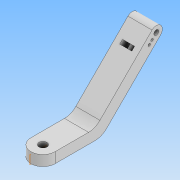
# Autodesk Inventor part: 主吊臂
Saved by Autodesk Inventor 2021 (Build 250183000, 183)
## iProperties
Created: 2025-12-12
Part Number: 主吊臂
Material: 一般
Document SubType Name: Modeling
Designer: User
Density: 1 g/cm^3
Appearance: 預設
Author: User
Autodesk Inventor part; units mm, degrees
ref_plane "YZ Plane" through (0, 0, 0) normal (1, 0, 0) x (0, 1, 0)
ref_plane "XZ Plane" through (0, 0, 0) normal (0, 1, 0) x (-1, 0, 0)
ref_plane "XY Plane" through (0, 0, 0) normal (0, 0, 1) x (1, 0, 0)
sketch "草圖1" plane through (0, 0, 0) normal (0, 1, 0) x (-1, 0, 0)
  line L0 (0, 150) -> (-300, 150)
  line L1 (-300, 0) -> (-300, 150)
  arc A0 (-300, 0) -> (0, 0) centre (-150, 0) ccw
  line L2 (0, 150) -> (0, 0)
  line L3 (0, 271.7864) -> (0, 150)
  line L4 (-300, 271.7864) -> (0, 271.7864)
  line L5 (-300, 150) -> (-300, 271.7864)
  circle A1 centre (-150, 0) radius 50
  line L6 (-30.3819, -276.523) -> (-200, -276.523)
  line L7 (0, -703.0461) -> (-300, -703.0461)
  line L8 (-300, -553.0461) -> (-300, -703.0461)
  arc A2 (0, -553.0461) -> (-300, -553.0461) centre (-150, -553.0461) ccw
  line L9 (0, -703.0461) -> (0, -553.0461)
  circle A3 centre (-150, -553.0461) radius 50
  constraints: 20 end point, 7 symmetric about line, 4 centre point, 4 point on circle, 1 horizontal, 2 other
extrude "擠出1" add sketch "草圖1" along normal blind 130 contours L7 L8 A2 L9
ref_plane "工作平面1" through (150, 0, -553.0461) normal (1, 0, 0) x (0, 0, -1)
sketch "草圖2" plane through (150, 0, -553.0461) normal (1, 0, 0) x (0, 0, -1)
  line L0 (-150, 0) -> (-150, 130) projected
  line L1 (-150, 130) -> (-50, 130) projected
  line L2 (-50, 130) -> (-50, 0) projected
  line L3 (-50, 0) -> (-150, 0) projected
  line L4 (150, 130) -> (150, 0) projected
  line L5 (150, 0) -> (50, 0) projected
  line L6 (50, 0) -> (50, 130) projected
  line L7 (50, 130) -> (150, 130) projected
  line L8 (150, 0) -> (150, 130) projected
  line L9 (150, 130) -> (500, 130)
  line L10 (500, 130) -> (500, 0)
  line L11 (500, 0) -> (150, 0)
  line L12 (150, 0) -> (150, 130)
  line L13 (150, 130) -> (0, 130) projected
  line L14 (500, 130) -> (606.066, 23.934)
  line L15 (606.066, 23.934) -> (1313.1728, 731.0408)
  line L16 (1313.1728, 731.0408) -> (1207.1068, 837.1068)
  line L17 (1207.1068, 837.1068) -> (500, 130)
  line L18 (606.066, 23.934) -> (582.132, 0)
  line L19 (500, 0) -> (582.132, 0)
  circle A0 centre (1260.1398, 784.0738) radius 75
  circle A1 centre (1207.1068, 731.0408) radius 15
  line L20 (1260.1398, 784.0738) -> (1207.1068, 731.0408)
  circle A2 centre (1260.1398, 784.0738) radius 30
  circle A3 centre (1171.7514, 695.6854) radius 15
  line L21 (1207.1068, 731.0408) -> (1171.7514, 695.6854)
  point P0 (-553.0461, 0)
  point P1 (1313.1728, 731.0408)
  dimension "d2" = 500
  dimension "d3" = 1000
  dimension "d4" = 150
  dimension "d5" = 45
  dimension "d6" = 30
  dimension "d7" = 60
  dimension "d8" = 30
  dimension "d9" = 50
  constraints: 24 end point, 5 parallel, 4 centre point, 2 collinear, 2 horizontal, 2 perpendicular, 2 point on circle, 1 coincident, 1 midpoint, 1 point on line, 1 tangent
  measures "d2" distance from line of L10 L13.end
  measures "d3" distance of L15.end L14.end
  measures "d4" distance of L9.end L14.end
  measures "d5" angle of L17 L9
  measures "d6" diameter of A1
  measures "d7" diameter of A2
  measures "d8" diameter of A3
  measures "d9" distance of L21.end L20.end
extrude "擠出2" add sketch "草圖2" along normal mid plane 300 contours L9 L10 L11 L4 | L14 L18 L19 L10 | L17 A0 A1 L15 L14 | A0 L16 A2 | L16 A2 L20 A1 A0 | A0 A1 L20 A2 L16
sketch "草圖3" plane through (0, 130, -1053.0461) normal (0, 0.7071, 0.7071) x (1, 0, 0)
  line L0 (0, -183.8478) -> (0, 0) projected
  line L1 (0, 0) -> (0, 1000) projected
  line L2 (0, 1000) -> (300, 1000) projected
  line L3 (300, 1000) -> (300, 0) projected
  line L4 (0, 0) -> (300, 0) projected
  line L5 (300, -183.8478) -> (0, -183.8478) projected
  line L6 (300, 0) -> (300, -183.8478) projected
  line L7 (75, 800) -> (225, 800)
  line L8 (225, 800) -> (225, 750)
  line L9 (225, 750) -> (75, 750)
  line L10 (75, 750) -> (75, 800)
  point P0 (0, -836.5399)
  point P1 (150, 800)
  point P2 (150, 1000)
  dimension "d12" = 200
  dimension "d13" = 50
  dimension "d14" = 150
  constraints: 8 end point, 2 midpoint, 2 parallel, 1 horizontal, 1 perpendicular, 1 vertical alignment
  measures "d12" distance between parallel lines of L2 L7
  measures "d13" distance of L7.end L8.end
  measures "d14" distance of L8.end L9.end
extrude "擠出3" cut sketch "草圖3" against normal blind 300 contours L7 L8 L9 L10
fillet "圓角1" radius 200 2 edges at (150, 130, -1053.0461) (150, 0, -1135.1781)
sketch "草圖4" plane through (225, 660.3301, -1583.3761) normal (0, 0.7071, -0.7071) x (-1, 0, 0)
  line L0 (225, -150) -> (150, -150) projected
  line L1 (150, -150) -> (0, -150) projected
  line L2 (0, -150) -> (-75, -150) projected
  line L3 (-75, -150) -> (-75, 0) projected
  line L4 (-75, 0) -> (0, 0) projected
  line L5 (0, 0) -> (0, -150) projected
  line L6 (225, 0) -> (225, -150) projected
  line L7 (150, 0) -> (225, 0) projected
  line L8 (0, 0) -> (150, 0) projected
  line L9 (150, -150) -> (150, 0) projected
  circle A0 centre (75, -75) radius 25
  point P0 (225, 652.6921)
  point P1 (75, 0)
  point P2 (0, -75)
  dimension "d18" = 50
  constraints: 2 midpoint, 1 centre point, 1 horizontal alignment, 1 vertical alignment
  measures "d18" diameter of A0
extrude "擠出4" add sketch "草圖4" along normal up to next contours A0
equation "\"d8\" = d6"
